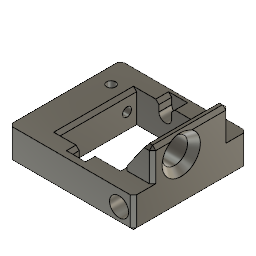
idler-roller (Autodesk Fusion 360 design; units mm, degrees)
Autodesk Fusion 360 part; units mm, degrees
note: some values were not read from the file. Set by a fixed rule: which sketch regions a step uses.
sketch "Sketch1" plane through (0, 0, 0) normal (0, 0, 1) x (1, 0, 0)
  line L0 (0, 0) -> (39, 0)
  line L1 (39, 0) -> (39, 35)
  line L2 (39, 35) -> (0, 35)
  line L3 (0, 35) -> (0, 0)
  line L4 (10, 30) -> (28, 30)
  line L5 (28, 30) -> (28, 5)
  line L6 (28, 5) -> (10, 5)
  line L7 (10, 5) -> (10, 30)
  dimension "d1" = 39
  dimension "d2" = 35
  dimension "d3" = 25
  dimension "d4" = 18
  dimension "d6" = 5
  dimension "d9" = 11
  measures "d1" distance of L0.start L0.end
  measures "d2" distance of L0.start L2.end
  measures "d3" distance of L4.end L5.end
  measures "d4" distance of L5 L7
  measures "d6" distance of L2 L4
  measures "d9" distance of L1 L5
extrude "Extrude1" add sketch "Sketch1" along normal blind 10
sketch "Sketch2" plane through (0, 0, 10) normal (0, 0, 1) x (-1, 0, 0)
  line L0 (-28, -5) -> (-10, -5)
  line L1 (-10, -5) -> (-10, -30)
  line L2 (-10, -30) -> (-28, -30)
  line L3 (-28, -30) -> (-28, -5)
  line L4 (0, -35) -> (0, 0)
  line L5 (0, 0) -> (-39, 0)
  line L6 (-39, 0) -> (-39, -35)
  line L7 (-39, -35) -> (0, -35)
  line L8 (-17, -34) -> (-21, -34)
  line L9 (-21, -34) -> (-21, -2)
  line L10 (-21, -2) -> (-17, -2)
  line L11 (-17, -2) -> (-17, -34)
  dimension "d10" = 32
  dimension "d11" = 4
  dimension "d12" = 7
  dimension "d49" = 1
  measures "d10" distance of L8.end L9.end
  measures "d11" distance of L9 L11
  measures "d12" distance of L2.end L9
  measures "d49" distance of L7 L8
extrude "Extrude2" cut sketch "Sketch2" against normal blind 5 contours L0 L9 L10 L11 | L0 L2 L9 L11 | L2 L8 L9 L11
fillet "Fillet1" radius 2 4 edges at (17, 32, 5) (21, 32, 5) (17, 3.5, 5) (21, 3.5, 5)
sketch "Sketch3" plane through (0, 35, 0) normal (0, 1, 0) x (-1, 0, 0)
  line L0 (-39, 0) -> (0, 0)
  line L1 (0, 0) -> (0, 10)
  line L2 (0, 10) -> (-39, 10)
  line L3 (-39, 10) -> (-39, 0)
  circle A0 centre (-34.5, 5) radius 1.75
  dimension "d16" = 3.5
  dimension "d17" = 5
  dimension "d21" = 4.5
  measures "d16" diameter of A0
  measures "d17" distance of L2 A0.centre
  measures "d21" distance of L3 A0.centre
extrude "Extrude3" cut sketch "Sketch3" against normal blind 36 contours A0
sketch "Sketch4" plane through (0, 35, 0) normal (0, 1, 0) x (-1, 0, 0)
  circle A0 centre (-34.5, 5) radius 1.75
  line L0 (-39, 0) -> (0, 0)
  line L1 (0, 0) -> (0, 10)
  line L2 (0, 10) -> (-39, 10)
  line L3 (-39, 10) -> (-39, 0)
  line L4 (-39, 10) -> (-30, 10)
  line L5 (-30, 10) -> (-30, 0)
  line L6 (-30, 0) -> (-39, 0)
  line L7 (-39, 0) -> (-39, 10)
extrude "Extrude4" add sketch "Sketch4" along normal blind 0.6 contours L0 L2 L3 L4 L5 L6 L7
sketch "Sketch5" plane through (0, 0, 0) normal (0, -1, 0) x (1, 0, 0)
  circle A0 centre (34.5, 5) radius 1.75
  line L0 (0, 0) -> (39, 0)
  line L1 (39, 0) -> (39, 10)
  line L2 (39, 10) -> (0, 10)
  line L3 (0, 10) -> (0, 0)
  circle A1 centre (34.5, 5) radius 3
  dimension "d24" = 6
  measures "d24" diameter of A1
extrude "Extrude5" cut sketch "Sketch5" against normal blind 11.6 contours A1
sketch "Sketch6" plane through (0, 0, 0) normal (-1, 0, 0) x (0, -1, 0)
  line L0 (-35, 0) -> (0, 0)
  line L1 (0, 0) -> (0, 10)
  line L2 (0, 10) -> (-35, 10)
  line L3 (-35, 10) -> (-35, 0)
  circle A0 centre (-27, 5) radius 1.4
  dimension "d28" = 2.8
  dimension "d30" = 8
  dimension "d32" = 5
  measures "d28" diameter of A0
  measures "d30" distance of L3 A0.centre
  measures "d32" distance of L0 A0.centre
extrude "Extrude6" cut sketch "Sketch6" against normal blind 10 contours A0
sketch "Sketch7" plane through (0, 0, 10) normal (0, 0, 1) x (-1, 0, 0)
  line L0 (-21, -34) -> (-21, -30)
  line L1 (-21, -30) -> (-28, -30)
  line L2 (-28, -30) -> (-28, -5)
  line L3 (-28, -5) -> (-21, -5)
  line L4 (-21, -5) -> (-21, -2)
  line L5 (-21, -2) -> (-17, -2)
  line L6 (-17, -2) -> (-17, -5)
  line L7 (-17, -5) -> (-10, -5)
  line L8 (-10, -5) -> (-10, -30)
  line L9 (-10, -30) -> (-17, -30)
  line L10 (-17, -30) -> (-17, -34)
  line L11 (-17, -34) -> (-21, -34)
  line L12 (0, -35) -> (0, 0)
  line L13 (0, 0) -> (-39, 0)
  line L14 (-39, 0) -> (-39, -35.6)
  line L15 (-39, -35.6) -> (-30, -35.6)
  line L16 (-30, -35.6) -> (-30, -35)
  line L17 (-30, -35) -> (0, -35)
  circle A0 centre (-5, -27) radius 1.4
  dimension "d35" = 2.8
  dimension "d36" = 8
  dimension "d37" = 5
  measures "d35" diameter of A0
  measures "d36" distance of L17 A0.centre
  measures "d37" distance of L12 A0.centre
extrude "Extrude7" cut sketch "Sketch7" against normal blind 12 contours A0
sketch "Sketch8" plane through (0, 0, 10) normal (0, 0, 1) x (-1, 0, 0)
  circle A0 centre (-5, -27) radius 1.4
  line L0 (-21, -34) -> (-21, -30)
  line L1 (-21, -30) -> (-28, -30)
  line L2 (-28, -30) -> (-28, -5)
  line L3 (-28, -5) -> (-21, -5)
  line L4 (-21, -5) -> (-21, -2)
  line L5 (-21, -2) -> (-17, -2)
  line L6 (-17, -2) -> (-17, -5)
  line L7 (-17, -5) -> (-10, -5)
  line L8 (-10, -5) -> (-10, -30)
  line L9 (-10, -30) -> (-17, -30)
  line L10 (-17, -30) -> (-17, -34)
  line L11 (-17, -34) -> (-21, -34)
  line L12 (0, -35) -> (0, 0)
  line L13 (0, 0) -> (-39, 0)
  line L14 (-39, 0) -> (-39, -35.6)
  line L15 (-39, -35.6) -> (-30, -35.6)
  line L16 (-30, -35.6) -> (-30, -35)
  line L17 (-30, -35) -> (0, -35)
  line L18 (-39, -6) -> (-30, -6)
  line L19 (-30, -6) -> (-30, -30)
  line L20 (-30, -30) -> (-39, -30)
  line L21 (-39, -30) -> (-39, -6)
extrude "Extrude8" add sketch "Sketch8" along normal blind 10 contours L14 L18 L19 L20 L21
sketch "Sketch9" plane through (39, 0, 0) normal (1, 0, 0) x (0, 1, 0)
  line L0 (0, 0) -> (35.6, 0)
  line L1 (35.6, 0) -> (35.6, 10)
  line L2 (35.6, 10) -> (30, 10)
  line L3 (30, 20) -> (6, 20)
  line L4 (0, 10) -> (0, 0)
  circle A0 centre (15, 14) radius 4
  line L5 (30, 10) -> (30, 20)
  line L6 (6, 20) -> (6, 10)
  line L7 (6, 10) -> (0, 10)
  dimension "d44" = 8
  dimension "d46" = 14
  dimension "d50" = 15
  measures "d44" diameter of A0
  measures "d46" distance of L0 A0.centre
  measures "d50" distance of L4 A0.centre
extrude "Extrude9" cut sketch "Sketch9" against normal blind 12 contours A0
chamfer "Chamfer2" distance 1 angle 45 20 edges at (10, 17.5, 10) (17, 32, 10) (21, 3.5, 10) (17, 3.5, 10) (21, 32, 10) (0, 0, 5) (0, 35, 5) (39, 0, 5) (39, 35.6, 5) (39, 30, 15) (30, 30, 15) (30, 6, 15) (39, 6, 15) (39, 18, 20) (34.5, 6, 20) (34.5, 30, 20) (15, 35, 0) (0, 17.5, 0) (19.5, 0, 0) (39, 17.8, 0)
chamfer "Chamfer3" distance 2 angle 45 1 edges at (39, 11.2707, 15.4465)
chamfer "Chamfer4" distance 7 distance2 10 1 edges at (30, 18, 20) measured on face at (35.3333, 14.3333, 20)
chamfer "Chamfer5" distance 2 angle 45 1 edges at (28, 17.5, 10)
